Autodesk Inventor part; units mm, degrees
(part 2 of 3)
sketch "Sketch36" plane through (-207.790264, 3.175, 44.45) normal (0, 1, 0) x (1, 0, 0)
  line L0 (58.565264, -107.95) -> (58.565264, 0)
  line L1 (58.565264, -53.975) -> (199.680527, -53.975) construction
  circle A0 centre (63.645264, -95.6945) radius 2.54
  line L2 (58.565264, 0) -> (58.565264, -107.95)
  line L3 (58.565264, -107.95) -> (0, -107.95)
  line L4 (0, -107.95) -> (0, -130.193109)
  line L5 (0, -130.193109) -> (56.388618, -144.290264)
  line L6 (56.388618, -144.290264) -> (84.727264, -144.290264)
  line L7 (84.727264, -144.290264) -> (84.727264, -141.115264)
  line L8 (84.727264, -141.115264) -> (68.090264, -141.115264)
  line L9 (68.090264, -141.115264) -> (68.090264, -130.320264)
  line L10 (68.090264, -130.320264) -> (84.727264, -130.320264)
  line L11 (84.727264, -130.320264) -> (84.727264, -120.160264)
  line L12 (84.727264, -120.160264) -> (102.253264, -120.160264)
  line L13 (102.253264, -120.160264) -> (102.253264, -130.320264)
  line L14 (102.253264, -130.320264) -> (118.890264, -130.320264)
  line L15 (118.890264, -130.320264) -> (118.890264, -141.115264)
  line L16 (118.890264, -141.115264) -> (102.253264, -141.115264)
  line L17 (102.253264, -141.115264) -> (102.253264, -144.290264)
  line L18 (102.253264, -144.290264) -> (199.680527, -144.290264)
  line L19 (199.680527, -144.290264) -> (199.680527, 36.340264)
  line L20 (199.680527, 36.340264) -> (102.253264, 36.340264)
  line L21 (102.253264, 36.340264) -> (102.253264, 33.165264)
  line L22 (102.253264, 33.165264) -> (118.890264, 33.165264)
  line L23 (118.890264, 33.165264) -> (118.890264, 22.370264)
  line L24 (118.890264, 22.370264) -> (102.253264, 22.370264)
  line L25 (102.253264, 22.370264) -> (102.253264, 12.210264)
  line L26 (102.253264, 12.210264) -> (84.727264, 12.210264)
  line L27 (84.727264, 12.210264) -> (84.727264, 22.370264)
  line L28 (84.727264, 22.370264) -> (68.090264, 22.370264)
  line L29 (68.090264, 22.370264) -> (68.090264, 33.165264)
  line L30 (68.090264, 33.165264) -> (84.727264, 33.165264)
  line L31 (84.727264, 33.165264) -> (84.727264, 36.340264)
  line L32 (84.727264, 36.340264) -> (56.388618, 36.340264)
  line L33 (56.388618, 36.340264) -> (36.467264, 31.359925)
  line L34 (36.467264, 31.359925) -> (36.467264, 24.13)
  line L35 (36.467264, 24.13) -> (7.547563, 24.13)
  line L36 (7.547563, 24.13) -> (0, 22.243109)
  line L37 (0, 22.243109) -> (0, 0)
  line L38 (0, 0) -> (58.565264, 0)
  circle A1 centre (128.542264, -12.2555) radius 2.54
  circle A2 centre (128.542264, -95.6945) radius 2.54
  circle A3 centre (63.645264, -12.2555) radius 2.54
  line L39 (133.005527, 33.165264) -> (183.805527, 33.165264)
  line L40 (183.805527, 33.165264) -> (183.805527, 11.575264)
  line L41 (183.805527, 11.575264) -> (133.005527, 11.575264)
  line L42 (133.005527, 11.575264) -> (133.005527, 33.165264)
  line L43 (133.005527, -119.525264) -> (183.805527, -119.525264)
  line L44 (183.805527, -119.525264) -> (183.805527, -141.115264)
  line L45 (183.805527, -141.115264) -> (133.005527, -141.115264)
  line L46 (133.005527, -141.115264) -> (133.005527, -119.525264)
  line L47 (144.892727, -46.336736) -> (144.892727, 9.670264)
  line L48 (144.892727, 9.670264) -> (185.532727, 9.670264)
  line L49 (185.532727, 9.670264) -> (185.532727, -46.336736)
  line L50 (185.532727, -46.336736) -> (144.892727, -46.336736)
  line L51 (144.892727, -117.620264) -> (144.892727, -61.613264)
  line L52 (144.892727, -61.613264) -> (185.532727, -61.613264)
  line L53 (185.532727, -61.613264) -> (185.532727, -117.620264)
  line L54 (185.532727, -117.620264) -> (144.892727, -117.620264)
  line L55 (63.645264, -53.975) -> (67.311438, -47.625)
  line L56 (67.311438, -47.625) -> (74.643786, -47.625)
  line L57 (74.643786, -47.625) -> (78.309961, -53.975)
  line L58 (78.309961, -53.975) -> (74.643786, -60.325)
  line L59 (74.643786, -60.325) -> (67.311438, -60.325)
  line L60 (67.311438, -60.325) -> (63.645264, -53.975)
  line L61 (79.043195, -62.865) -> (82.70937, -56.515)
  line L62 (82.70937, -56.515) -> (90.041718, -56.515)
  line L63 (90.041718, -56.515) -> (93.707892, -62.865)
  line L64 (93.707892, -62.865) -> (90.041718, -69.215)
  line L65 (90.041718, -69.215) -> (82.70937, -69.215)
  line L66 (82.70937, -69.215) -> (79.043195, -62.865)
  line L67 (82.70937, -51.435) -> (79.043195, -45.085)
  line L68 (90.041718, -51.435) -> (82.70937, -51.435)
  line L69 (79.043195, -45.085) -> (82.70937, -38.735)
  line L70 (93.707892, -45.085) -> (90.041718, -51.435)
  line L71 (82.70937, -38.735) -> (90.041718, -38.735)
  line L72 (90.041718, -38.735) -> (93.707892, -45.085)
  line L73 (67.311438, -78.105) -> (63.645264, -71.755)
  line L74 (74.643786, -78.105) -> (67.311438, -78.105)
  line L75 (63.645264, -71.755) -> (67.311438, -65.405)
  line L76 (78.309961, -71.755) -> (74.643786, -78.105)
  line L77 (67.311438, -65.405) -> (74.643786, -65.405)
  line L78 (74.643786, -65.405) -> (78.309961, -71.755)
  line L79 (79.043195, -9.525) -> (82.70937, -3.175)
  line L80 (82.70937, -3.175) -> (90.041718, -3.175)
  line L81 (74.643786, -12.065) -> (78.309961, -18.415)
  line L82 (82.70937, -15.875) -> (79.043195, -9.525)
  line L83 (90.041718, -15.875) -> (82.70937, -15.875)
  line L84 (93.707892, -9.525) -> (90.041718, -15.875)
  line L85 (90.041718, -3.175) -> (93.707892, -9.525)
  line L86 (78.309961, -36.195) -> (74.643786, -42.545)
  line L87 (74.643786, -42.545) -> (67.311438, -42.545)
  line L88 (67.311438, -42.545) -> (63.645264, -36.195)
  line L89 (63.645264, -18.415) -> (67.311438, -12.065)
  line L90 (67.311438, -12.065) -> (74.643786, -12.065)
  line L91 (78.309961, -18.415) -> (74.643786, -24.765)
  line L92 (82.70937, -20.955) -> (90.041718, -20.955)
  line L93 (79.043195, -27.305) -> (82.70937, -20.955)
  line L94 (90.041718, -20.955) -> (93.707892, -27.305)
  line L95 (93.707892, -27.305) -> (90.041718, -33.655)
  line L96 (90.041718, -33.655) -> (82.70937, -33.655)
  line L97 (74.643786, -24.765) -> (67.311438, -24.765)
  line L98 (67.311438, -24.765) -> (63.645264, -18.415)
  line L99 (82.70937, -33.655) -> (79.043195, -27.305)
  line L100 (67.311438, -29.845) -> (74.643786, -29.845)
  line L101 (74.643786, -29.845) -> (78.309961, -36.195)
  line L102 (63.645264, -36.195) -> (67.311438, -29.845)
  line L103 (109.523195, -45.085) -> (113.18937, -38.735)
  line L104 (113.18937, -38.735) -> (120.521718, -38.735)
  line L105 (105.123786, -47.625) -> (108.789961, -53.975)
  line L106 (113.18937, -51.435) -> (109.523195, -45.085)
  line L107 (120.521718, -51.435) -> (113.18937, -51.435)
  line L108 (124.187892, -45.085) -> (120.521718, -51.435)
  line L109 (120.521718, -38.735) -> (124.187892, -45.085)
  line L110 (108.789961, -71.755) -> (105.123786, -78.105)
  line L111 (105.123786, -78.105) -> (97.791438, -78.105)
  line L112 (97.791438, -78.105) -> (94.125264, -71.755)
  line L113 (94.125264, -53.975) -> (97.791438, -47.625)
  line L114 (97.791438, -47.625) -> (105.123786, -47.625)
  line L115 (108.789961, -53.975) -> (105.123786, -60.325)
  line L116 (113.18937, -56.515) -> (120.521718, -56.515)
  line L117 (109.523195, -62.865) -> (113.18937, -56.515)
  line L118 (120.521718, -56.515) -> (124.187892, -62.865)
  line L119 (124.187892, -62.865) -> (120.521718, -69.215)
  line L120 (120.521718, -69.215) -> (113.18937, -69.215)
  line L121 (105.123786, -60.325) -> (97.791438, -60.325)
  line L122 (97.791438, -60.325) -> (94.125264, -53.975)
  line L123 (113.18937, -69.215) -> (109.523195, -62.865)
  line L124 (97.791438, -65.405) -> (105.123786, -65.405)
  line L125 (105.123786, -65.405) -> (108.789961, -71.755)
  line L126 (94.125264, -71.755) -> (97.791438, -65.405)
  line L127 (109.523195, -9.525) -> (113.18937, -3.175)
  line L128 (113.18937, -3.175) -> (120.521718, -3.175)
  line L129 (105.123786, -12.065) -> (108.789961, -18.415)
  line L130 (113.18937, -15.875) -> (109.523195, -9.525)
  line L131 (120.521718, -15.875) -> (113.18937, -15.875)
  line L132 (124.187892, -9.525) -> (120.521718, -15.875)
  line L133 (120.521718, -3.175) -> (124.187892, -9.525)
  line L134 (108.789961, -36.195) -> (105.123786, -42.545)
  line L135 (105.123786, -42.545) -> (97.791438, -42.545)
  line L136 (97.791438, -42.545) -> (94.125264, -36.195)
  line L137 (94.125264, -18.415) -> (97.791438, -12.065)
  line L138 (97.791438, -12.065) -> (105.123786, -12.065)
  line L139 (108.789961, -18.415) -> (105.123786, -24.765)
  line L140 (113.18937, -20.955) -> (120.521718, -20.955)
  line L141 (109.523195, -27.305) -> (113.18937, -20.955)
  line L142 (120.521718, -20.955) -> (124.187892, -27.305)
  line L143 (124.187892, -27.305) -> (120.521718, -33.655)
  line L144 (120.521718, -33.655) -> (113.18937, -33.655)
  line L145 (105.123786, -24.765) -> (97.791438, -24.765)
  line L146 (97.791438, -24.765) -> (94.125264, -18.415)
  line L147 (113.18937, -33.655) -> (109.523195, -27.305)
  line L148 (97.791438, -29.845) -> (105.123786, -29.845)
  line L149 (105.123786, -29.845) -> (108.789961, -36.195)
  line L150 (94.125264, -36.195) -> (97.791438, -29.845)
  line L151 (140.003195, -45.085) -> (143.66937, -38.735)
  line L152 (143.66937, -38.735) -> (151.001718, -38.735)
  line L153 (135.603786, -47.625) -> (139.269961, -53.975)
  line L154 (143.66937, -51.435) -> (140.003195, -45.085)
  line L155 (151.001718, -51.435) -> (143.66937, -51.435)
  line L156 (154.667892, -45.085) -> (151.001718, -51.435)
  line L157 (151.001718, -38.735) -> (154.667892, -45.085)
  line L158 (139.269961, -71.755) -> (135.603786, -78.105)
  line L159 (135.603786, -78.105) -> (128.271438, -78.105)
  line L160 (128.271438, -78.105) -> (124.605264, -71.755)
  line L161 (124.605264, -53.975) -> (128.271438, -47.625)
  line L162 (128.271438, -47.625) -> (135.603786, -47.625)
  line L163 (139.269961, -53.975) -> (135.603786, -60.325)
  line L164 (143.66937, -56.515) -> (151.001718, -56.515)
  line L165 (140.003195, -62.865) -> (143.66937, -56.515)
  line L166 (151.001718, -56.515) -> (154.667892, -62.865)
  line L167 (154.667892, -62.865) -> (151.001718, -69.215)
  line L168 (151.001718, -69.215) -> (143.66937, -69.215)
  line L169 (135.603786, -60.325) -> (128.271438, -60.325)
  line L170 (128.271438, -60.325) -> (124.605264, -53.975)
  line L171 (143.66937, -69.215) -> (140.003195, -62.865)
  line L172 (128.271438, -65.405) -> (135.603786, -65.405)
  line L173 (135.603786, -65.405) -> (139.269961, -71.755)
  line L174 (124.605264, -71.755) -> (128.271438, -65.405)
  line L175 (140.003195, -9.525) -> (143.66937, -3.175)
  line L176 (143.66937, -3.175) -> (151.001718, -3.175)
  line L177 (135.603786, -12.065) -> (139.269961, -18.415)
  line L178 (143.66937, -15.875) -> (140.003195, -9.525)
  line L179 (151.001718, -15.875) -> (143.66937, -15.875)
  line L180 (154.667892, -9.525) -> (151.001718, -15.875)
  line L181 (151.001718, -3.175) -> (154.667892, -9.525)
  line L182 (139.269961, -36.195) -> (135.603786, -42.545)
  line L183 (135.603786, -42.545) -> (128.271438, -42.545)
  line L184 (128.271438, -42.545) -> (124.605264, -36.195)
  line L185 (124.605264, -18.415) -> (128.271438, -12.065)
  line L186 (128.271438, -12.065) -> (135.603786, -12.065)
  line L187 (139.269961, -18.415) -> (135.603786, -24.765)
  line L188 (143.66937, -20.955) -> (151.001718, -20.955)
  line L189 (140.003195, -27.305) -> (143.66937, -20.955)
  line L190 (151.001718, -20.955) -> (154.667892, -27.305)
  line L191 (154.667892, -27.305) -> (151.001718, -33.655)
  line L192 (151.001718, -33.655) -> (143.66937, -33.655)
  line L193 (135.603786, -24.765) -> (128.271438, -24.765)
  line L194 (128.271438, -24.765) -> (124.605264, -18.415)
  line L195 (143.66937, -33.655) -> (140.003195, -27.305)
  line L196 (128.271438, -29.845) -> (135.603786, -29.845)
  line L197 (135.603786, -29.845) -> (139.269961, -36.195)
  line L198 (124.605264, -36.195) -> (128.271438, -29.845)
  line L199 (124.187892, -80.645) -> (120.521718, -86.995)
  line L200 (128.271438, -95.885) -> (124.605264, -89.535)
  line L201 (135.603786, -95.885) -> (128.271438, -95.885)
  line L202 (128.271438, -83.185) -> (135.603786, -83.185)
  line L203 (139.269961, -89.535) -> (135.603786, -95.885)
  line L204 (135.603786, -83.185) -> (139.269961, -89.535)
  line L205 (124.605264, -89.535) -> (128.271438, -83.185)
  line L206 (74.643786, -95.885) -> (67.311438, -95.885)
  line L207 (78.309961, -89.535) -> (74.643786, -95.885)
  line L208 (67.311438, -95.885) -> (63.645264, -89.535)
  line L209 (74.643786, -83.185) -> (78.309961, -89.535)
  line L210 (63.645264, -89.535) -> (67.311438, -83.185)
  line L211 (67.311438, -83.185) -> (74.643786, -83.185)
  line L212 (82.70937, -86.995) -> (79.043195, -80.645)
  line L213 (90.041718, -86.995) -> (82.70937, -86.995)
  line L214 (97.791438, -95.885) -> (94.125264, -89.535)
  line L215 (93.707892, -80.645) -> (90.041718, -86.995)
  line L216 (97.791438, -83.185) -> (105.123786, -83.185)
  line L217 (94.125264, -89.535) -> (97.791438, -83.185)
  line L218 (120.521718, -86.995) -> (113.18937, -86.995)
  line L219 (113.18937, -86.995) -> (109.523195, -80.645)
  line L220 (105.123786, -83.185) -> (108.789961, -89.535)
  line L221 (108.789961, -89.535) -> (105.123786, -95.885)
  line L222 (105.123786, -95.885) -> (97.791438, -95.885)
  line L223 (120.521718, -74.295) -> (124.187892, -80.645)
  line L224 (113.18937, -74.295) -> (120.521718, -74.295)
  line L225 (109.523195, -80.645) -> (113.18937, -74.295)
  line L226 (82.70937, -74.295) -> (90.041718, -74.295)
  line L227 (90.041718, -74.295) -> (93.707892, -80.645)
  line L228 (79.043195, -80.645) -> (82.70937, -74.295)
  line L229 (124.187892, -98.425) -> (120.521718, -104.775)
  line L230 (128.271438, -113.665) -> (124.605264, -107.315)
  line L231 (135.603786, -113.665) -> (128.271438, -113.665)
  line L232 (128.271438, -100.965) -> (135.603786, -100.965)
  line L233 (139.269961, -107.315) -> (135.603786, -113.665)
  line L234 (135.603786, -100.965) -> (139.269961, -107.315)
  line L235 (124.605264, -107.315) -> (128.271438, -100.965)
  line L236 (74.643786, -113.665) -> (67.311438, -113.665)
  line L237 (78.309961, -107.315) -> (74.643786, -113.665)
  line L238 (67.311438, -113.665) -> (63.645264, -107.315)
  line L239 (74.643786, -100.965) -> (78.309961, -107.315)
  line L240 (63.645264, -107.315) -> (67.311438, -100.965)
  line L241 (67.311438, -100.965) -> (74.643786, -100.965)
  line L242 (82.70937, -104.775) -> (79.043195, -98.425)
  line L243 (90.041718, -104.775) -> (82.70937, -104.775)
  line L244 (97.791438, -113.665) -> (94.125264, -107.315)
  line L245 (93.707892, -98.425) -> (90.041718, -104.775)
  line L246 (97.791438, -100.965) -> (105.123786, -100.965)
  line L247 (94.125264, -107.315) -> (97.791438, -100.965)
  line L248 (120.521718, -104.775) -> (113.18937, -104.775)
  line L249 (113.18937, -104.775) -> (109.523195, -98.425)
  line L250 (105.123786, -100.965) -> (108.789961, -107.315)
  line L251 (108.789961, -107.315) -> (105.123786, -113.665)
  line L252 (105.123786, -113.665) -> (97.791438, -113.665)
  line L253 (120.521718, -92.075) -> (124.187892, -98.425)
  line L254 (113.18937, -92.075) -> (120.521718, -92.075)
  line L255 (109.523195, -98.425) -> (113.18937, -92.075)
  line L256 (82.70937, -92.075) -> (90.041718, -92.075)
  line L257 (90.041718, -92.075) -> (93.707892, -98.425)
  line L258 (79.043195, -98.425) -> (82.70937, -92.075)
  line L259 (67.311438, -6.985) -> (63.645264, -0.635)
  line L260 (63.645264, -0.635) -> (67.311438, 5.715)
  line L261 (74.643786, -6.985) -> (67.311438, -6.985)
  line L262 (67.311438, 5.715) -> (74.643786, 5.715)
  line L263 (74.643786, 5.715) -> (78.309961, -0.635)
  line L264 (78.309961, -0.635) -> (74.643786, -6.985)
  line L265 (98.107301, -6.985) -> (94.441127, -0.635)
  line L266 (94.441127, -0.635) -> (98.107301, 5.715)
  line L267 (105.43965, -6.985) -> (98.107301, -6.985)
  line L268 (98.107301, 5.715) -> (105.43965, 5.715)
  line L269 (105.43965, 5.715) -> (109.105824, -0.635)
  line L270 (109.105824, -0.635) -> (105.43965, -6.985)
  line L271 (128.587301, -6.985) -> (124.921127, -0.635)
  line L272 (124.921127, -0.635) -> (128.587301, 5.715)
  line L273 (135.91965, -6.985) -> (128.587301, -6.985)
  line L274 (128.587301, 5.715) -> (135.91965, 5.715)
  line L275 (135.91965, 5.715) -> (139.585824, -0.635)
  line L276 (139.585824, -0.635) -> (135.91965, -6.985)
  point P0 (207.790264, 44.45)
  point P1 (70.977612, -53.975)
  point P2 (86.375544, -62.865)
  point P3 (86.375544, -45.085)
  point P4 (70.977612, -71.755)
  point P5 (86.375544, -9.525)
  point P6 (70.977612, -36.195)
  point P7 (70.977612, -18.415)
  point P8 (86.375544, -27.305)
  point P9 (116.855544, -45.085)
  point P10 (101.457612, -71.755)
  point P11 (101.457612, -53.975)
  point P12 (116.855544, -62.865)
  point P13 (116.855544, -9.525)
  point P14 (101.457612, -36.195)
  point P15 (101.457612, -18.415)
  point P16 (116.855544, -27.305)
  point P17 (147.335544, -45.085)
  point P18 (131.937612, -71.755)
  point P19 (131.937612, -53.975)
  point P20 (147.335544, -62.865)
  point P21 (147.335544, -9.525)
  point P22 (131.937612, -36.195)
  point P23 (131.937612, -18.415)
  point P24 (147.335544, -27.305)
  point P25 (131.937612, -89.535)
  point P26 (70.977612, -89.535)
  point P27 (101.457612, -89.535)
  point P28 (116.855544, -80.645)
  point P29 (86.375544, -80.645)
  point P30 (131.937612, -107.315)
  point P31 (70.977612, -107.315)
  point P32 (101.457612, -107.315)
  point P33 (116.855544, -98.425)
  point P34 (86.375544, -98.425)
  point P35 (70.977612, -0.635)
  point P36 (101.773476, -0.635)
  point P37 (132.253476, -0.635)
  dimension "d309" = 12.7
  dimension "d310" = 12.7
  dimension "d311" = 5.08
  dimension "d312" = 12.7
  dimension "d313" = 5.08
  dimension "d314" = 5.08
  dimension "d315" = 12.7
  dimension "d316" = 5.08
  dimension "d317" = 5.08
  dimension "d318" = 5.08
  dimension "d321" = 35.56
  dimension "d324" = 30.48
  dimension "d329" = 17.78
  dimension "d334" = 12.7
  dimension "d335" = 12.7
  dimension "d336" = 12.7
  dimension "d337" = 5.08
  dimension "d338" = 5.08
  dimension "d339" = 5.08
  dimension "d340" = 5.08
  dimension "d341" = 5.08
  dimension "d342" = 5.08
  constraints: 446 end point, 2 horizontal, 2 midpoint, 2 point on line, 2 vertical, 1 vertical alignment, 481 other
  measures "d309" distance between parallel lines of L60 L57
  measures "d310" distance between parallel lines of L66 L63
  measures "d311" distance between parallel lines of L58 L61
  measures "d312" distance between parallel lines of L67 L72
  measures "d313" distance between parallel lines of L57 L67
  measures "d314" distance between parallel lines of L62 L68
  measures "d315" distance between parallel lines of L73 L78
  measures "d316" distance between parallel lines of L66 L78
  measures "d317" distance between parallel lines of L59 L77
  measures "d318" distance from line of L0 L55.start
  measures "d321" distance of L69.end L79.end
  measures "d324" distance of L69.end L103.end
  measures "d329" distance of L118.end L199.start
  measures "d334" distance between parallel lines of L259 L263
  measures "d335" distance between parallel lines of L265 L269
  measures "d336" distance between parallel lines of L271 L275
  measures "d337" distance between parallel lines of L90 L261
  measures "d338" distance between parallel lines of L79 L264
  measures "d339" distance between parallel lines of L85 L265
  measures "d340" distance between parallel lines of L138 L267
  measures "d341" distance between parallel lines of L133 L271
  measures "d342" distance between parallel lines of L186 L273
extrude "Cutouts1" cut sketch "Sketch36" against normal blind 25.4 contours L55 L56 L57 L58 L59 L60 | L61 L62 L63 L64 L65 L66 | L67 L69 L71 L72 L70 L68 | L73 L75 L77 L78 L76 L74 | L79 L80 L85 L84 L83 L82 | L86 L87 L88 L102 L100 L101 | L92 L94 L95 L96 L99 L93 | L103 L104 L109 L108 L107 L106 | L105 L115 L121 L122 L113 L114 | L110 L111 L112 L126 L124 L125 | L116 L118 L119 L120 L123 L117 | L127 L128 L133 L132 L131 L130 | L129 L139 L145 L146 L137 L138 | L134 L135 L136 L150 L148 L149 | L140 L142 L143 L144 L147 L141 | L153 L163 L169 L170 L161 L162 | L158 L159 L160 L174 L172 L173 | L182 L183 L184 L198 L196 L197 | L199 L218 L219 L225 L224 L223 | L212 L228 L226 L227 L215 L213 | L214 L217 L216 L220 L221 L222 | L229 L248 L249 L255 L254 L253 | L230 L235 L232 L234 L233 L231 | L236 L238 L240 L241 L239 L237 | L242 L258 L256 L257 L245 L243 | L244 L247 L246 L250 L251 L252 | L259 L260 L262 L263 L264 L261 | L265 L266 L268 L269 L270 L267 | L271 L272 L274 L275 L276 L273
sketch "Sketch37" plane through (-207.790264, 3.175, 44.45) normal (0, 1, 0) x (1, 0, 0)
  circle A0 centre (128.542264, -12.2555) radius 2.54
  circle A1 centre (128.542264, -95.6945) radius 2.54
  circle A2 centre (63.645264, -12.2555) radius 2.54
  circle A3 centre (63.645264, -95.6945) radius 2.54
  line L0 (36.467264, 24.13) -> (7.547563, 24.13)
  line L1 (7.547563, 24.13) -> (0, 22.243109)
  line L2 (0, 22.243109) -> (0, 0)
  line L3 (0, 0) -> (58.565264, 0)
  line L4 (58.565264, 0) -> (58.565264, -107.95)
  line L5 (58.565264, -107.95) -> (0, -107.95)
  line L6 (0, -107.95) -> (0, -130.193109)
  line L7 (0, -130.193109) -> (56.388618, -144.290264)
  line L8 (56.388618, -144.290264) -> (84.727264, -144.290264)
  line L9 (84.727264, -144.290264) -> (84.727264, -141.115264)
  line L10 (84.727264, -141.115264) -> (68.090264, -141.115264)
  line L11 (68.090264, -141.115264) -> (68.090264, -130.320264)
  line L12 (68.090264, -130.320264) -> (84.727264, -130.320264)
  line L13 (84.727264, -130.320264) -> (84.727264, -120.160264)
  line L14 (84.727264, -120.160264) -> (102.253264, -120.160264)
  line L15 (102.253264, -120.160264) -> (102.253264, -130.320264)
  line L16 (102.253264, -130.320264) -> (118.890264, -130.320264)
  line L17 (118.890264, -130.320264) -> (118.890264, -141.115264)
  line L18 (118.890264, -141.115264) -> (102.253264, -141.115264)
  line L19 (102.253264, -141.115264) -> (102.253264, -144.290264)
  line L20 (102.253264, -144.290264) -> (199.680527, -144.290264)
  line L21 (199.680527, -144.290264) -> (199.680527, 36.340264)
  line L22 (199.680527, 36.340264) -> (102.253264, 36.340264)
  line L23 (102.253264, 36.340264) -> (102.253264, 33.165264)
  line L24 (102.253264, 33.165264) -> (118.890264, 33.165264)
  line L25 (118.890264, 33.165264) -> (118.890264, 22.370264)
  line L26 (118.890264, 22.370264) -> (102.253264, 22.370264)
  line L27 (102.253264, 22.370264) -> (102.253264, 12.210264)
  line L28 (102.253264, 12.210264) -> (84.727264, 12.210264)
  line L29 (84.727264, 12.210264) -> (84.727264, 22.370264)
  line L30 (84.727264, 22.370264) -> (68.090264, 22.370264)
  line L31 (68.090264, 22.370264) -> (68.090264, 33.165264)
  line L32 (68.090264, 33.165264) -> (84.727264, 33.165264)
  line L33 (84.727264, 33.165264) -> (84.727264, 36.340264)
  line L34 (84.727264, 36.340264) -> (56.388618, 36.340264)
  line L35 (56.388618, 36.340264) -> (36.467264, 31.359925)
  line L36 (36.467264, 31.359925) -> (36.467264, 24.13)
  line L37 (144.892727, -117.620264) -> (144.892727, -61.613264)
  line L38 (144.892727, -61.613264) -> (185.532727, -61.613264)
  line L39 (185.532727, -61.613264) -> (185.532727, -117.620264)
  line L40 (185.532727, -117.620264) -> (144.892727, -117.620264)
  line L41 (144.892727, -46.336736) -> (144.892727, 9.670264)
  line L42 (144.892727, 9.670264) -> (185.532727, 9.670264)
  line L43 (185.532727, 9.670264) -> (185.532727, -46.336736)
  line L44 (185.532727, -46.336736) -> (144.892727, -46.336736)
  line L45 (133.005527, -119.525264) -> (183.805527, -119.525264)
  line L46 (183.805527, -119.525264) -> (183.805527, -141.115264)
  line L47 (183.805527, -141.115264) -> (133.005527, -141.115264)
  line L48 (133.005527, -141.115264) -> (133.005527, -119.525264)
  line L49 (133.005527, 33.165264) -> (183.805527, 33.165264)
  line L50 (183.805527, 33.165264) -> (183.805527, 11.575264)
  line L51 (183.805527, 11.575264) -> (133.005527, 11.575264)
  line L52 (133.005527, 11.575264) -> (133.005527, 33.165264)
  line L53 (192.606627, -144.290264) -> (192.606627, 36.340264) construction
  line L54 (193.241627, 22.225) -> (191.654127, 19.475369)
  line L55 (191.654127, 19.475369) -> (188.479127, 19.475369)
  line L56 (188.479127, 19.475369) -> (186.891627, 22.225)
  line L57 (186.891627, 22.225) -> (188.479127, 24.974631)
  line L58 (188.479127, 24.974631) -> (191.654127, 24.974631)
  line L59 (191.654127, 24.974631) -> (193.241627, 22.225)
  line L60 (193.559127, 25.825369) -> (191.971627, 28.575)
  line L61 (191.971627, 28.575) -> (193.559127, 31.324631)
  line L62 (193.559127, 31.324631) -> (196.734127, 31.324631)
  line L63 (196.734127, 31.324631) -> (198.321627, 28.575)
  line L64 (198.321627, 28.575) -> (196.734127, 25.825369)
  line L65 (196.734127, 25.825369) -> (193.559127, 25.825369)
  line L66 (192.606627, -156.990264) -> (192.606627, 23.640264) construction
  line L67 (191.654127, 6.775369) -> (188.479127, 6.775369)
  line L68 (193.241627, 9.525) -> (191.654127, 6.775369)
  line L69 (188.479127, 6.775369) -> (186.891627, 9.525)
  line L70 (186.891627, 9.525) -> (188.479127, 12.274631)
  line L71 (188.479127, 12.274631) -> (191.654127, 12.274631)
  line L72 (196.734127, 13.125369) -> (193.559127, 13.125369)
  line L73 (198.321627, 15.875) -> (196.734127, 13.125369)
  line L74 (193.559127, 13.125369) -> (191.971627, 15.875)
  line L75 (196.734127, 18.624631) -> (198.321627, 15.875)
  line L76 (191.971627, 15.875) -> (193.559127, 18.624631)
  line L77 (193.559127, 18.624631) -> (196.734127, 18.624631)
  line L78 (191.654127, 12.274631) -> (193.241627, 9.525)
  line L79 (192.606627, -169.690264) -> (192.606627, 10.940264) construction
  line L80 (191.654127, -5.924631) -> (188.479127, -5.924631)
  line L81 (193.241627, -3.175) -> (191.654127, -5.924631)
  line L82 (188.479127, -5.924631) -> (186.891627, -3.175)
  line L83 (186.891627, -3.175) -> (188.479127, -0.425369)
  line L84 (188.479127, -0.425369) -> (191.654127, -0.425369)
  line L85 (196.734127, 0.425369) -> (193.559127, 0.425369)
  line L86 (198.321627, 3.175) -> (196.734127, 0.425369)
  line L87 (193.559127, 0.425369) -> (191.971627, 3.175)
  line L88 (196.734127, 5.924631) -> (198.321627, 3.175)
  line L89 (191.971627, 3.175) -> (193.559127, 5.924631)
  line L90 (193.559127, 5.924631) -> (196.734127, 5.924631)
  line L91 (191.654127, -0.425369) -> (193.241627, -3.175)
  line L92 (192.606627, -182.390264) -> (192.606627, -1.759736) construction
  line L93 (191.654127, -18.624631) -> (188.479127, -18.624631)
  line L94 (193.241627, -15.875) -> (191.654127, -18.624631)
  line L95 (188.479127, -18.624631) -> (186.891627, -15.875)
  line L96 (186.891627, -15.875) -> (188.479127, -13.125369)
  line L97 (188.479127, -13.125369) -> (191.654127, -13.125369)
  line L98 (196.734127, -12.274631) -> (193.559127, -12.274631)
  line L99 (198.321627, -9.525) -> (196.734127, -12.274631)
  line L100 (193.559127, -12.274631) -> (191.971627, -9.525)
  line L101 (196.734127, -6.775369) -> (198.321627, -9.525)
  line L102 (191.971627, -9.525) -> (193.559127, -6.775369)
  line L103 (193.559127, -6.775369) -> (196.734127, -6.775369)
  line L104 (191.654127, -13.125369) -> (193.241627, -15.875)
  line L105 (192.606627, -195.090264) -> (192.606627, -14.459736) construction
  line L106 (191.654127, -31.324631) -> (188.479127, -31.324631)
  line L107 (193.241627, -28.575) -> (191.654127, -31.324631)
  line L108 (188.479127, -31.324631) -> (186.891627, -28.575)
  line L109 (186.891627, -28.575) -> (188.479127, -25.825369)
  line L110 (188.479127, -25.825369) -> (191.654127, -25.825369)
  line L111 (196.734127, -24.974631) -> (193.559127, -24.974631)
  line L112 (198.321627, -22.225) -> (196.734127, -24.974631)
  line L113 (193.559127, -24.974631) -> (191.971627, -22.225)
  line L114 (196.734127, -19.475369) -> (198.321627, -22.225)
  line L115 (191.971627, -22.225) -> (193.559127, -19.475369)
  line L116 (193.559127, -19.475369) -> (196.734127, -19.475369)
  line L117 (191.654127, -25.825369) -> (193.241627, -28.575)
  line L118 (192.606627, -207.790264) -> (192.606627, -27.159736) construction
  line L119 (191.654127, -44.024631) -> (188.479127, -44.024631)
  line L120 (193.241627, -41.275) -> (191.654127, -44.024631)
  line L121 (188.479127, -44.024631) -> (186.891627, -41.275)
  line L122 (186.891627, -41.275) -> (188.479127, -38.525369)
  line L123 (188.479127, -38.525369) -> (191.654127, -38.525369)
  line L124 (196.734127, -37.674631) -> (193.559127, -37.674631)
  line L125 (198.321627, -34.925) -> (196.734127, -37.674631)
  line L126 (193.559127, -37.674631) -> (191.971627, -34.925)
  line L127 (196.734127, -32.175369) -> (198.321627, -34.925)
  line L128 (191.971627, -34.925) -> (193.559127, -32.175369)
  line L129 (193.559127, -32.175369) -> (196.734127, -32.175369)
  line L130 (191.654127, -38.525369) -> (193.241627, -41.275)
  line L131 (192.606627, -220.490264) -> (192.606627, -39.859736) construction
  line L132 (191.654127, -56.724631) -> (188.479127, -56.724631)
  line L133 (193.241627, -53.975) -> (191.654127, -56.724631)
  line L134 (188.479127, -56.724631) -> (186.891627, -53.975)
  line L135 (186.891627, -53.975) -> (188.479127, -51.225369)
  line L136 (188.479127, -51.225369) -> (191.654127, -51.225369)
  line L137 (196.734127, -50.374631) -> (193.559127, -50.374631)
  line L138 (198.321627, -47.625) -> (196.734127, -50.374631)
  line L139 (193.559127, -50.374631) -> (191.971627, -47.625)
  line L140 (196.734127, -44.875369) -> (198.321627, -47.625)
  line L141 (191.971627, -47.625) -> (193.559127, -44.875369)
  line L142 (193.559127, -44.875369) -> (196.734127, -44.875369)
  line L143 (191.654127, -51.225369) -> (193.241627, -53.975)
  line L144 (192.606627, -233.190264) -> (192.606627, -52.559736) construction
  line L145 (191.654127, -69.424631) -> (188.479127, -69.424631)
  line L146 (193.241627, -66.675) -> (191.654127, -69.424631)
  line L147 (188.479127, -69.424631) -> (186.891627, -66.675)
  line L148 (186.891627, -66.675) -> (188.479127, -63.925369)
  line L149 (188.479127, -63.925369) -> (191.654127, -63.925369)
  line L150 (196.734127, -63.074631) -> (193.559127, -63.074631)
  line L151 (198.321627, -60.325) -> (196.734127, -63.074631)
  line L152 (193.559127, -63.074631) -> (191.971627, -60.325)
  line L153 (196.734127, -57.575369) -> (198.321627, -60.325)
  line L154 (191.971627, -60.325) -> (193.559127, -57.575369)
  line L155 (193.559127, -57.575369) -> (196.734127, -57.575369)
  line L156 (191.654127, -63.925369) -> (193.241627, -66.675)
  line L157 (192.606627, -245.890264) -> (192.606627, -65.259736) construction
  line L158 (191.654127, -82.124631) -> (188.479127, -82.124631)
  line L159 (193.241627, -79.375) -> (191.654127, -82.124631)
  line L160 (188.479127, -82.124631) -> (186.891627, -79.375)
  line L161 (186.891627, -79.375) -> (188.479127, -76.625369)
  line L162 (188.479127, -76.625369) -> (191.654127, -76.625369)
  line L163 (196.734127, -75.774631) -> (193.559127, -75.774631)
  line L164 (198.321627, -73.025) -> (196.734127, -75.774631)
  line L165 (193.559127, -75.774631) -> (191.971627, -73.025)
  line L166 (196.734127, -70.275369) -> (198.321627, -73.025)
  line L167 (191.971627, -73.025) -> (193.559127, -70.275369)
  line L168 (193.559127, -70.275369) -> (196.734127, -70.275369)
  line L169 (191.654127, -76.625369) -> (193.241627, -79.375)
  line L170 (192.606627, -258.590264) -> (192.606627, -77.959736) construction
  line L171 (191.654127, -94.824631) -> (188.479127, -94.824631)
  line L172 (193.241627, -92.075) -> (191.654127, -94.824631)
  line L173 (188.479127, -94.824631) -> (186.891627, -92.075)
  line L174 (186.891627, -92.075) -> (188.479127, -89.325369)
  line L175 (188.479127, -89.325369) -> (191.654127, -89.325369)
  line L176 (196.734127, -88.474631) -> (193.559127, -88.474631)
  line L177 (198.321627, -85.725) -> (196.734127, -88.474631)
  line L178 (193.559127, -88.474631) -> (191.971627, -85.725)
  line L179 (196.734127, -82.975369) -> (198.321627, -85.725)
  line L180 (191.971627, -85.725) -> (193.559127, -82.975369)
  line L181 (193.559127, -82.975369) -> (196.734127, -82.975369)
  line L182 (191.654127, -89.325369) -> (193.241627, -92.075)
  line L183 (192.606627, -271.290264) -> (192.606627, -90.659736) construction
  line L184 (191.654127, -107.524631) -> (188.479127, -107.524631)
  line L185 (193.241627, -104.775) -> (191.654127, -107.524631)
  line L186 (188.479127, -107.524631) -> (186.891627, -104.775)
  line L187 (186.891627, -104.775) -> (188.479127, -102.025369)
  line L188 (188.479127, -102.025369) -> (191.654127, -102.025369)
  line L189 (196.734127, -101.174631) -> (193.559127, -101.174631)
  line L190 (198.321627, -98.425) -> (196.734127, -101.174631)
  line L191 (193.559127, -101.174631) -> (191.971627, -98.425)
  line L192 (196.734127, -95.675369) -> (198.321627, -98.425)
  line L193 (191.971627, -98.425) -> (193.559127, -95.675369)
  line L194 (193.559127, -95.675369) -> (196.734127, -95.675369)
  line L195 (191.654127, -102.025369) -> (193.241627, -104.775)
  line L196 (192.606627, -283.990264) -> (192.606627, -103.359736) construction
  line L197 (191.654127, -120.224631) -> (188.479127, -120.224631)
  line L198 (193.241627, -117.475) -> (191.654127, -120.224631)
  line L199 (188.479127, -120.224631) -> (186.891627, -117.475)
  line L200 (186.891627, -117.475) -> (188.479127, -114.725369)
  line L201 (188.479127, -114.725369) -> (191.654127, -114.725369)
  line L202 (196.734127, -113.874631) -> (193.559127, -113.874631)
  line L203 (198.321627, -111.125) -> (196.734127, -113.874631)
  line L204 (193.559127, -113.874631) -> (191.971627, -111.125)
  line L205 (196.734127, -108.375369) -> (198.321627, -111.125)
  line L206 (191.971627, -111.125) -> (193.559127, -108.375369)
  line L207 (193.559127, -108.375369) -> (196.734127, -108.375369)
  line L208 (191.654127, -114.725369) -> (193.241627, -117.475)
  line L209 (192.606627, -296.690264) -> (192.606627, -116.059736) construction
  line L210 (191.654127, -132.924631) -> (188.479127, -132.924631)
  line L211 (193.241627, -130.175) -> (191.654127, -132.924631)
  line L212 (188.479127, -132.924631) -> (186.891627, -130.175)
  line L213 (186.891627, -130.175) -> (188.479127, -127.425369)
  line L214 (188.479127, -127.425369) -> (191.654127, -127.425369)
  line L215 (196.734127, -126.574631) -> (193.559127, -126.574631)
  line L216 (198.321627, -123.825) -> (196.734127, -126.574631)
  line L217 (193.559127, -126.574631) -> (191.971627, -123.825)
  line L218 (196.734127, -121.075369) -> (198.321627, -123.825)
  line L219 (191.971627, -123.825) -> (193.559127, -121.075369)
  line L220 (193.559127, -121.075369) -> (196.734127, -121.075369)
  line L221 (191.654127, -127.425369) -> (193.241627, -130.175)
  line L222 (58.565264, -53.975) -> (199.680527, -53.975) construction
  line L223 (193.559127, -139.274631) -> (191.971627, -136.525)
  line L224 (191.971627, -136.525) -> (193.559127, -133.775369)
  line L225 (193.559127, -133.775369) -> (196.734127, -133.775369)
  line L226 (196.734127, -133.775369) -> (198.321627, -136.525)
  line L227 (198.321627, -136.525) -> (196.734127, -139.274631)
  line L228 (196.734127, -139.274631) -> (193.559127, -139.274631)
  point P0 (207.790264, 44.45)
  point P1 (190.066627, 22.225)
  point P2 (195.146627, 28.575)
  point P3 (190.066627, 9.525)
  point P4 (195.146627, 15.875)
  point P5 (190.066627, -3.175)
  point P6 (195.146627, 3.175)
  point P7 (190.066627, -15.875)
  point P8 (195.146627, -9.525)
  point P9 (190.066627, -28.575)
  point P10 (195.146627, -22.225)
  point P11 (190.066627, -41.275)
  point P12 (195.146627, -34.925)
  point P13 (190.066627, -53.975)
  point P14 (195.146627, -47.625)
  point P15 (190.066627, -66.675)
  point P16 (195.146627, -60.325)
  point P17 (190.066627, -79.375)
  point P18 (195.146627, -73.025)
  point P19 (190.066627, -92.075)
  point P20 (195.146627, -85.725)
  point P21 (190.066627, -104.775)
  point P22 (195.146627, -98.425)
  point P23 (190.066627, -117.475)
  point P24 (195.146627, -111.125)
  point P25 (190.066627, -130.175)
  point P26 (195.146627, -123.825)
  point P27 (195.146627, -136.525)
  dimension "d345" = 7.0739
  dimension "d347" = 3.175
  dimension "d349" = 2.54
  dimension "d350" = 2.54
  dimension "d353" = 12.7
  dimension "d359" = 6.35
  dimension "d360" = 6.35
  constraints: 352 end point, 3 horizontal, 3 point on line, 2 equal length, 2 midpoint, 2 vertical, 1 perpendicular, 1 vertical alignment, 387 other
  measures "d345" distance between parallel lines of L53 L21
  measures "d347" distance of L54.end L55.end
  measures "d349" distance from line of L53 point (190.067, 22.225)
  measures "d350" distance from line of L53 point (195.147, 28.575)
  measures "d353" distance of L53.start L66.start
  measures "d359" vertical distance of point (195.147, 28.575) point (190.067, 22.225)
  measures "d360" vertical distance of point (190.067, -130.175) point (195.147, -136.525)
extrude "Cutouts2" cut sketch "Sketch37" against normal up to next contours L54 L55 L56 L57 L58 L59 | L60 L61 L62 L63 L64 L65 | L67 L69 L70 L71 L78 L68 | L72 L74 L76 L77 L75 L73 | L80 L82 L83 L84 L91 L81 | L85 L87 L89 L90 L88 L86 | L93 L95 L96 L97 L104 L94 | L98 L100 L102 L103 L101 L99 | L106 L108 L109 L110 L117 L107 | L111 L113 L115 L116 L114 L112 | L119 L121 L122 L123 L130 L120 | L124 L126 L128 L129 L127 L125 | L132 L134 L135 L136 L143 L133 | L137 L139 L141 L142 L140 L138 | L145 L147 L148 L149 L156 L146 | L150 L152 L154 L155 L153 L151 | L158 L160 L161 L162 L169 L159 | L163 L165 L167 L168 L166 L164 | L171 L173 L174 L175 L182 L172 | L176 L178 L180 L181 L179 L177 | L184 L186 L187 L188 L195 L185 | L189 L191 L193 L194 L192 L190 | L197 L199 L200 L201 L208 L198 | L202 L204 L206 L207 L205 L203 | L210 L212 L213 L214 L221 L211 | L215 L217 L219 L220 L218 L216 | L223 L224 L225 L226 L227 L228
sketch "Sketch39" plane through (-152.4, 0, 47.625) normal (-1, 0, 0) x (0, 0, 1)
  line L0 (-3.175, 3.175) -> (104.775, 3.175)
  line L1 (0, 0) -> (101.6, 0)
  line L2 (101.6, 0) -> (101.6, 50.8)
  line L3 (0, 50.8) -> (101.6, 50.8)
  line L4 (0, 0) -> (0, 50.8)
  line L5 (50.8, 50.8) -> (50.8, 3.175) construction
  line L6 (4.7625, 5.207) -> (11.1125, 5.207)
  line L7 (11.1125, 5.207) -> (7.9375, 10.706261)
  line L8 (7.9375, 10.706261) -> (4.7625, 5.207)
  line L9 (14.2875, 5.207) -> (20.6375, 5.207)
  line L10 (20.6375, 5.207) -> (17.4625, 10.706261)
  line L11 (17.4625, 10.706261) -> (14.2875, 5.207)
  line L12 (23.8125, 5.207) -> (30.1625, 5.207)
  line L13 (30.1625, 5.207) -> (26.9875, 10.706261)
  line L14 (26.9875, 10.706261) -> (23.8125, 5.207)
  line L15 (33.3375, 5.207) -> (39.6875, 5.207)
  line L16 (39.6875, 5.207) -> (36.5125, 10.706261)
  line L17 (36.5125, 10.706261) -> (33.3375, 5.207)
  line L18 (42.8625, 5.207) -> (49.2125, 5.207)
  line L19 (49.2125, 5.207) -> (46.0375, 10.706261)
  line L20 (46.0375, 10.706261) -> (42.8625, 5.207)
  line L21 (52.3875, 5.207) -> (58.7375, 5.207)
  line L22 (58.7375, 5.207) -> (55.5625, 10.706261)
  line L23 (55.5625, 10.706261) -> (52.3875, 5.207)
  line L24 (61.9125, 5.207) -> (68.2625, 5.207)
  line L25 (68.2625, 5.207) -> (65.0875, 10.706261)
  line L26 (65.0875, 10.706261) -> (61.9125, 5.207)
  line L27 (71.4375, 5.207) -> (77.7875, 5.207)
  line L28 (77.7875, 5.207) -> (74.6125, 10.706261)
  line L29 (74.6125, 10.706261) -> (71.4375, 5.207)
  line L30 (80.9625, 5.207) -> (87.3125, 5.207)
  line L31 (87.3125, 5.207) -> (84.1375, 10.706261)
  line L32 (84.1375, 10.706261) -> (80.9625, 5.207)
  line L33 (90.4875, 5.207) -> (96.8375, 5.207)
  line L34 (96.8375, 5.207) -> (93.6625, 10.706261)
  line L35 (93.6625, 10.706261) -> (90.4875, 5.207)
  line L36 (4.7625, 14.732) -> (11.1125, 14.732)
  line L37 (11.1125, 14.732) -> (7.9375, 20.231261)
  line L38 (7.9375, 20.231261) -> (4.7625, 14.732)
  line L39 (14.2875, 14.732) -> (20.6375, 14.732)
  line L40 (20.6375, 14.732) -> (17.4625, 20.231261)
  line L41 (17.4625, 20.231261) -> (14.2875, 14.732)
  line L42 (23.8125, 14.732) -> (30.1625, 14.732)
  line L43 (30.1625, 14.732) -> (26.9875, 20.231261)
  line L44 (26.9875, 20.231261) -> (23.8125, 14.732)
  line L45 (33.3375, 14.732) -> (39.6875, 14.732)
  line L46 (39.6875, 14.732) -> (36.5125, 20.231261)
  line L47 (36.5125, 20.231261) -> (33.3375, 14.732)
  line L48 (42.8625, 14.732) -> (49.2125, 14.732)
  line L49 (49.2125, 14.732) -> (46.0375, 20.231261)
  line L50 (46.0375, 20.231261) -> (42.8625, 14.732)
  line L51 (52.3875, 14.732) -> (58.7375, 14.732)
  line L52 (58.7375, 14.732) -> (55.5625, 20.231261)
  line L53 (55.5625, 20.231261) -> (52.3875, 14.732)
  line L54 (61.9125, 14.732) -> (68.2625, 14.732)
  line L55 (68.2625, 14.732) -> (65.0875, 20.231261)
  line L56 (65.0875, 20.231261) -> (61.9125, 14.732)
  line L57 (71.4375, 14.732) -> (77.7875, 14.732)
  line L58 (77.7875, 14.732) -> (74.6125, 20.231261)
  line L59 (74.6125, 20.231261) -> (71.4375, 14.732)
  line L60 (80.9625, 14.732) -> (87.3125, 14.732)
  line L61 (87.3125, 14.732) -> (84.1375, 20.231261)
  line L62 (84.1375, 20.231261) -> (80.9625, 14.732)
  line L63 (90.4875, 14.732) -> (96.8375, 14.732)
  line L64 (96.8375, 14.732) -> (93.6625, 20.231261)
  line L65 (93.6625, 20.231261) -> (90.4875, 14.732)
  line L66 (4.7625, 24.257) -> (11.1125, 24.257)
  line L67 (11.1125, 24.257) -> (7.9375, 29.756261)
  line L68 (7.9375, 29.756261) -> (4.7625, 24.257)
  line L69 (14.2875, 24.257) -> (20.6375, 24.257)
  line L70 (20.6375, 24.257) -> (17.4625, 29.756261)
  line L71 (17.4625, 29.756261) -> (14.2875, 24.257)
  line L72 (23.8125, 24.257) -> (30.1625, 24.257)
  line L73 (30.1625, 24.257) -> (26.9875, 29.756261)
  line L74 (26.9875, 29.756261) -> (23.8125, 24.257)
  line L75 (33.3375, 24.257) -> (39.6875, 24.257)
  line L76 (39.6875, 24.257) -> (36.5125, 29.756261)
  line L77 (36.5125, 29.756261) -> (33.3375, 24.257)
  line L78 (42.8625, 24.257) -> (49.2125, 24.257)
  line L79 (49.2125, 24.257) -> (46.0375, 29.756261)
  line L80 (46.0375, 29.756261) -> (42.8625, 24.257)
  line L81 (52.3875, 24.257) -> (58.7375, 24.257)
  line L82 (58.7375, 24.257) -> (55.5625, 29.756261)
  line L83 (55.5625, 29.756261) -> (52.3875, 24.257)
  line L84 (61.9125, 24.257) -> (68.2625, 24.257)
  line L85 (68.2625, 24.257) -> (65.0875, 29.756261)
  line L86 (65.0875, 29.756261) -> (61.9125, 24.257)
  line L87 (71.4375, 24.257) -> (77.7875, 24.257)
  line L88 (77.7875, 24.257) -> (74.6125, 29.756261)
  line L89 (74.6125, 29.756261) -> (71.4375, 24.257)
  line L90 (80.9625, 24.257) -> (87.3125, 24.257)
  line L91 (87.3125, 24.257) -> (84.1375, 29.756261)
  line L92 (84.1375, 29.756261) -> (80.9625, 24.257)
  line L93 (90.4875, 24.257) -> (96.8375, 24.257)
  line L94 (96.8375, 24.257) -> (93.6625, 29.756261)
  line L95 (93.6625, 29.756261) -> (90.4875, 24.257)
  line L96 (4.7625, 33.782) -> (11.1125, 33.782)
  line L97 (11.1125, 33.782) -> (7.9375, 39.281261)
  line L98 (7.9375, 39.281261) -> (4.7625, 33.782)
  line L99 (14.2875, 33.782) -> (20.6375, 33.782)
  line L100 (20.6375, 33.782) -> (17.4625, 39.281261)
  line L101 (17.4625, 39.281261) -> (14.2875, 33.782)
  line L102 (23.8125, 33.782) -> (30.1625, 33.782)
  line L103 (30.1625, 33.782) -> (26.9875, 39.281261)
  line L104 (26.9875, 39.281261) -> (23.8125, 33.782)
  line L105 (33.3375, 33.782) -> (39.6875, 33.782)
  line L106 (39.6875, 33.782) -> (36.5125, 39.281261)
  line L107 (36.5125, 39.281261) -> (33.3375, 33.782)
  line L108 (42.8625, 33.782) -> (49.2125, 33.782)
  line L109 (49.2125, 33.782) -> (46.0375, 39.281261)
  line L110 (46.0375, 39.281261) -> (42.8625, 33.782)
  line L111 (52.3875, 33.782) -> (58.7375, 33.782)
  line L112 (58.7375, 33.782) -> (55.5625, 39.281261)
  line L113 (55.5625, 39.281261) -> (52.3875, 33.782)
  line L114 (61.9125, 33.782) -> (68.2625, 33.782)
  line L115 (68.2625, 33.782) -> (65.0875, 39.281261)
  line L116 (65.0875, 39.281261) -> (61.9125, 33.782)
  line L117 (71.4375, 33.782) -> (77.7875, 33.782)
  line L118 (77.7875, 33.782) -> (74.6125, 39.281261)
  line L119 (74.6125, 39.281261) -> (71.4375, 33.782)
  line L120 (80.9625, 33.782) -> (87.3125, 33.782)
  line L121 (87.3125, 33.782) -> (84.1375, 39.281261)
  line L122 (84.1375, 39.281261) -> (80.9625, 33.782)
  line L123 (90.4875, 33.782) -> (96.8375, 33.782)
  line L124 (96.8375, 33.782) -> (93.6625, 39.281261)
  line L125 (93.6625, 39.281261) -> (90.4875, 33.782)
  line L126 (4.7625, 43.307) -> (11.1125, 43.307)
  line L127 (11.1125, 43.307) -> (7.9375, 48.806261)
  line L128 (7.9375, 48.806261) -> (4.7625, 43.307)
  line L129 (14.2875, 43.307) -> (20.6375, 43.307)
  line L130 (20.6375, 43.307) -> (17.4625, 48.806261)
  line L131 (17.4625, 48.806261) -> (14.2875, 43.307)
  line L132 (23.8125, 43.307) -> (30.1625, 43.307)
  line L133 (30.1625, 43.307) -> (26.9875, 48.806261)
  line L134 (26.9875, 48.806261) -> (23.8125, 43.307)
  line L135 (33.3375, 43.307) -> (39.6875, 43.307)
  line L136 (39.6875, 43.307) -> (36.5125, 48.806261)
  line L137 (36.5125, 48.806261) -> (33.3375, 43.307)
  line L138 (42.8625, 43.307) -> (49.2125, 43.307)
  line L139 (49.2125, 43.307) -> (46.0375, 48.806261)
  line L140 (46.0375, 48.806261) -> (42.8625, 43.307)
  line L141 (52.3875, 43.307) -> (58.7375, 43.307)
  line L142 (58.7375, 43.307) -> (55.5625, 48.806261)
  line L143 (55.5625, 48.806261) -> (52.3875, 43.307)
  line L144 (61.9125, 43.307) -> (68.2625, 43.307)
  line L145 (68.2625, 43.307) -> (65.0875, 48.806261)
  line L146 (65.0875, 48.806261) -> (61.9125, 43.307)
  line L147 (71.4375, 43.307) -> (77.7875, 43.307)
  line L148 (77.7875, 43.307) -> (74.6125, 48.806261)
  line L149 (74.6125, 48.806261) -> (71.4375, 43.307)
  line L150 (80.9625, 43.307) -> (87.3125, 43.307)
  line L151 (87.3125, 43.307) -> (84.1375, 48.806261)
  line L152 (84.1375, 48.806261) -> (80.9625, 43.307)
  line L153 (90.4875, 43.307) -> (96.8375, 43.307)
  line L154 (96.8375, 43.307) -> (93.6625, 48.806261)
  line L155 (93.6625, 48.806261) -> (90.4875, 43.307)
  line L156 (-3.175, 47.625) -> (104.775, 47.625)
  line L157 (-1.5875, 47.625) -> (-3.175, 47.625)
  line L158 (-1.5875, 47.625) -> (103.1875, 47.625)
  line L159 (104.775, 47.625) -> (103.1875, 47.625)
  line L160 (101.6, 0) -> (101.6, 50.8)
  line L161 (101.6, 46.0375) -> (0, 46.0375)
  point P0 (-47.625, 0)
  point P1 (101.6, 3.175)
  point P2 (0, 3.175)
  point P3 (28.586045, 46.0375)
  point P4 (25.388955, 46.0375)
  point P5 (38.111045, 46.0375)
  point P6 (34.913955, 46.0375)
  point P7 (57.161045, 46.0375)
  point P8 (53.963955, 46.0375)
  point P9 (76.211045, 46.0375)
  point P10 (73.013955, 46.0375)
  point P11 (95.261045, 46.0375)
  point P12 (92.063955, 46.0375)
  point P13 (19.061045, 46.0375)
  point P14 (15.863955, 46.0375)
  point P15 (47.636045, 46.0375)
  point P16 (44.438955, 46.0375)
  point P17 (66.686045, 46.0375)
  point P18 (63.488955, 46.0375)
  point P19 (85.736045, 46.0375)
  point P20 (82.538955, 46.0375)
  point P21 (9.536045, 46.0375)
  point P22 (6.338955, 46.0375)
  dimension "d369" = 60
  dimension "d370" = 6.35
  dimension "d373" = 9.525
  dimension "d376" = 9.525
  dimension "d379" = 1.5875
  dimension "d380" = 2.032
  dimension "d383" = 1.5875
  constraints: 302 end point, 2 horizontal, 2 midpoint, 2 point on line, 1 equal length, 1 vertical, 297 other
  measures "d369" angle of L7 L8
  measures "d370" distance of L6.start L6.end
  measures "d373" distance of L6.start L9.start
  measures "d376" distance of L6.start L36.start
  measures "d379" distance from line of L5 L141.start
  measures "d380" distance between parallel lines of L0 L18
extrude "Cutouts3" cut sketch "Sketch39" against normal up to surface (3.175 mm away) contours L0 L2 L1 L4 | L161 L127 L126 L128 | L154 L153 L155 L161 | L161 L130 L129 L131 | L151 L150 L152 L161 | L161 L133 L132 L134 | L148 L147 L149 L161 | L161 L136 L135 L137 | L145 L144 L146 L161 | L161 L139 L138 L140 | L142 L141 L143 L161 | L8 L7 L6 | L11 L10 L9 | L14 L13 L12 | L17 L16 L15 | L20 L19 L18 | L23 L22 L21 | L26 L25 L24 | L29 L28 L27 | L32 L31 L30 | L35 L34 L33 | L38 L37 L36 | L41 L40 L39 | L44 L43 L42 | L47 L46 L45 | L50 L49 L48 | L53 L52 L51 | L56 L55 L54 | L59 L58 L57 | L62 L61 L60 | L65 L64 L63 | L68 L67 L66 | L71 L70 L69 | L74 L73 L72 | L77 L76 L75 | L80 L79 L78 | L83 L82 L81 | L86 L85 L84 | L89 L88 L87 | L92 L91 L90 | L95 L94 L93 | L98 L97 L96 | L101 L100 L99 | L104 L103 L102 | L107 L106 L105 | L110 L109 L108 | L113 L112 L111 | L116 L115 L114 | L119 L118 L117 | L122 L121 L120 | L125 L124 L123